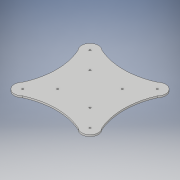
# Autodesk Inventor part: Base1
Saved by Autodesk Inventor 2019 (Build 230136000, 136)
## iProperties
Created: 2023-04-14
Part Number: Base1
Material: Generic
Document SubType Name: Modeling
Designer: Analuam
Density: 1 g/cm^3
Appearance: Default
Author: Analuam
Autodesk Inventor part; units mm, degrees
ref_plane "YZ Plane" through (0, 0, 0) normal (1, 0, 0) x (0, 1, 0)
ref_plane "XZ Plane" through (0, 0, 0) normal (0, 1, 0) x (-1, 0, 0)
ref_plane "XY Plane" through (0, 0, 0) normal (0, 0, 1) x (1, 0, 0)
sketch "Sketch1" plane through (0, 0, 0) normal (0, 1, 0) x (-1, 0, 0)
  arc A0 (-10.6066, -130.6066) -> (10.6066, -109.3934) centre (0, -120) ccw
  arc A1 (10.6066, -10.6066) -> (-10.6066, 10.6066) centre (0, 0) ccw
  arc A2 (-130.6066, -109.3934) -> (-109.3934, -130.6066) centre (-120, -120) ccw
  arc A3 (-109.3934, 10.6066) -> (-130.6066, -10.6066) centre (-120, 0) ccw
  arc A4 (10.6066, -10.6066) -> (10.6066, -109.3934) centre (120.3122, -60) ccw
  arc A5 (-10.6066, -130.6066) -> (-109.3934, -130.6066) centre (-60, -240.3122) ccw
  arc A6 (-109.3934, 10.6066) -> (-10.6066, 10.6066) centre (-60, 120.3122) ccw
  arc A7 (-130.6066, -109.3934) -> (-130.6066, -10.6066) centre (-244.217, -60) ccw
  circle A8 centre (0, 0) radius 1.5
  circle A9 centre (-31.0935, -31.0935) radius 1.5
  circle A10 centre (-88.9065, -31.0935) radius 1.5
  circle A11 centre (-88.9065, -88.9065) radius 1.5
  circle A12 centre (-31.0935, -88.9065) radius 1.5
  circle A13 centre (-120, 0) radius 1.5
  circle A14 centre (-120, -120) radius 1.5
  circle A15 centre (0, -120) radius 1.5
  point P0 (-60, -60)
  dimension "d36" = 360
  dimension "d40" = 360
  constraints: 16 centre point, 16 point on circle, 2 coincident, 18 other
sketch "Sketch3" plane through (0, 0, 0) normal (0, 1, 0) x (-1, 0, 0)
  circle A0 centre (-7.1, -120) radius 1
  point P0 (0, 0)
  constraints: 1 centre point
extrude "Extrusion1" add sketch "Sketch1" along normal blind 3
body "Solid1"
